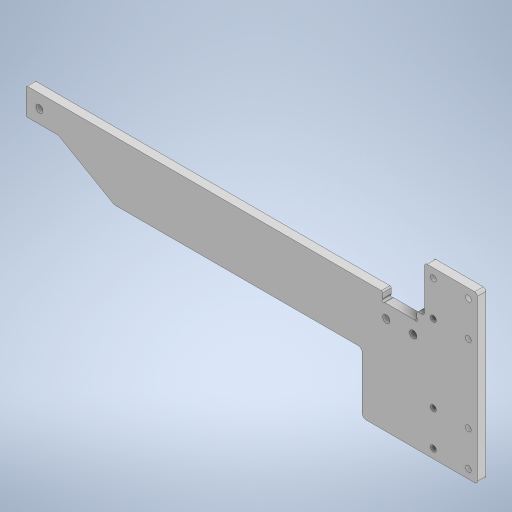
# Autodesk Inventor part: Z-Axis Bed Plates
Saved by Autodesk Inventor 2024 (Build 280153000, 153)
## iProperties
Created: 2024-08-02
Part Number: Z-Axis Bed Plates
Material: Generic
Document SubType Name: Modeling
Designer: Ishaan
Density: 1 g/cm^3
Appearance: Default
Author: Ishaan
Autodesk Inventor part; units mm, degrees
ref_plane "YZ Plane" through (0, 0, 0) normal (1, 0, 0) x (0, 1, 0)
ref_plane "XZ Plane" through (0, 0, 0) normal (0, 1, 0) x (-1, 0, 0)
sketch "Sketch1" plane through (0, 0, 0) normal (0, 0, 1) x (1, 0, 0)
  line L0 (19.7, -72.5) -> (-19.7, -72.5)
  line L1 (-19.7, -72.5) -> (-19.7, 72.5)
  line L2 (-19.7, 72.5) -> (19.7, 72.5)
  line L3 (19.7, 72.5) -> (19.7, -72.5)
  line L4 (19.7, -72.5) -> (-19.7, 72.5) construction
  line L5 (-19.7, -72.5) -> (19.7, 72.5) construction
  line L6 (19.7, 11.1) -> (-19.7, 11.1) construction
  line L7 (-19.7, 11.1) -> (-19.7, 72.5) construction
  line L8 (-19.7, 72.5) -> (19.7, 72.5) construction
  line L9 (19.7, 72.5) -> (19.7, 11.1) construction
  line L10 (19.7, 11.1) -> (-19.7, 72.5) construction
  line L11 (-19.7, 11.1) -> (19.7, 72.5) construction
  line L12 (19.7, -72.5) -> (-19.7, -72.5) construction
  line L13 (-19.7, -72.5) -> (-19.7, -11.1) construction
  line L14 (-19.7, -11.1) -> (19.7, -11.1) construction
  line L15 (19.7, -11.1) -> (19.7, -72.5) construction
  line L16 (19.7, -72.5) -> (-19.7, -11.1) construction
  line L17 (-19.7, -72.5) -> (19.7, -11.1) construction
  line L18 (19.7, 22.1) -> (-19.7, 22.1) construction
  line L19 (-19.7, 22.1) -> (-19.7, 61.5) construction
  line L20 (-19.7, 61.5) -> (19.7, 61.5)
  line L21 (19.7, 61.5) -> (19.7, 22.1) construction
  line L22 (19.7, 22.1) -> (-19.7, 61.5) construction
  line L23 (-19.7, 22.1) -> (19.7, 61.5) construction
  line L24 (19.7, -61.5) -> (-19.7, -61.5)
  line L25 (-19.7, -61.5) -> (-19.7, -22.1) construction
  line L26 (-19.7, -22.1) -> (19.7, -22.1) construction
  line L27 (19.7, -22.1) -> (19.7, -61.5) construction
  line L28 (19.7, -61.5) -> (-19.7, -22.1) construction
  line L29 (-19.7, -61.5) -> (19.7, -22.1) construction
  line L30 (13, 28.8) -> (-13, 28.8) construction
  line L31 (-13, 28.8) -> (-13, 54.8) construction
  line L32 (-13, 54.8) -> (13, 54.8) construction
  line L33 (13, 54.8) -> (13, 28.8) construction
  line L34 (13, 28.8) -> (-13, 54.8) construction
  line L35 (-13, 28.8) -> (13, 54.8) construction
  line L36 (13, -54.8) -> (-13, -54.8) construction
  line L37 (-13, -54.8) -> (-13, -28.8) construction
  line L38 (-13, -28.8) -> (13, -28.8) construction
  line L39 (13, -28.8) -> (13, -54.8) construction
  line L40 (13, -54.8) -> (-13, -28.8) construction
  line L41 (-13, -54.8) -> (13, -28.8) construction
  line L42 (-316, 27.5) -> (-19.7, 27.5)
  line L43 (-19.7, 27.5) -> (-19.7, 7.5)
  line L44 (-19.7, 7.5) -> (-316, 7.5)
  line L45 (-316, 7.5) -> (-316, 27.5)
  line L46 (19.7, -63.5) -> (19.7, -63.5)
  line L47 (19.772, 73.498) -> (19.772, 73.498)
  point P0 (0, 0)
  point P1 (0, 41.8)
  point P2 (0, -41.8)
  point P3 (-316, 17.5)
  point P4 (-291, 7.5)
  point P5 (17, 72.5)
  point P6 (17, -72.5)
  point P7 (-19.7, 27.5)
  point P8 (-19.7, 7.5)
  point P9 (-19.7, -61.5)
  point P10 (19.7, -61.5)
  dimension "d1" = 145
  dimension "d2" = 61.4
  dimension "d3" = 39.4
  dimension "d4" = 26
  dimension "d5" = 26
  dimension "d6" = 20
  dimension "d8" = 316
  dimension "d11" = 25
  dimension "d55" = 45
  dimension "d126" = 6.7
  dimension "d128" = 6.7
  constraints: 96 end point, 17 parallel, 15 midpoint, 9 collinear, 9 horizontal, 8 coincident, 8 perpendicular, 4 equal length, 2 point on line
  measures "d1" distance between parallel lines of L2 L0
  measures "d2" distance of L6.end L7.end
  measures "d3" distance of L18.end L19.end
  measures "d4" distance of L31.end L32.end
  measures "d5" distance of L30.end L31.end
  measures "d6" distance of L44.end L42.start
  measures "d8" distance from line of point (0, 41.8) L45
  measures "d11" distance from line of point (-291, 7.5) L45
  measures "d55" distance between parallel lines of L2 L42
  measures "d126" distance from line of L20 point (13, 54.8)
  measures "d128" distance between parallel lines of L21 L33
extrude "Extrusion1" add sketch "Sketch1" along normal blind 6.35 contours L24 L1 L20 L3 | L44 L45 L42 L1
sketch "Sketch2" plane through (0, 0, 6.35) normal (0, 0, 1) x (1, 0, 0)
  line L0 (19.7, -61.5) -> (19.7, 61.5) projected
  line L1 (-19.7, 61.5) -> (-19.7, 27.5) projected
  line L2 (-19.7, 27.5) -> (-316, 27.5) projected
  line L3 (-316, 27.5) -> (-316, 7.5) projected
  line L4 (-316, 7.5) -> (-19.7, 7.5) projected
  line L5 (-19.7, 7.5) -> (-19.7, -61.5) projected
  line L6 (19.7, -61.5) -> (-19.7, -61.5) construction
  line L7 (-19.7, -61.5) -> (19.7, -61.5) projected
  line L8 (19.7, 61.5) -> (-19.7, 61.5) projected
  line L9 (-19.7, -61.5) -> (-66, -61.5)
  line L10 (-66, -16.5) -> (-250.4308, -16.5)
  line L11 (-250.4308, -16.5) -> (-292, 7.5)
  line L12 (-66, -16.5) -> (-66, -61.5)
  point P0 (0, 0)
  point P1 (0, 41.8)
  point P2 (0, -41.8)
  point P3 (13, 28.8)
  point P4 (13, -28.8)
  dimension "d25" = 24
  dimension "d124" = 34
  dimension "d140" = 24
  dimension "d142" = 85.7
  dimension "d143" = 150
  constraints: 8 end point, 2 horizontal, 2 point on line, 1 collinear, 1 parallel
  measures "d25" distance from line of L11.end L3
  measures "d124" distance between parallel lines of L8 L2
  measures "d140" distance between parallel lines of L10 L4
  measures "d142" distance from line of L0 L9.end
  measures "d143" angle of L10 L11
extrude "Extrusion2" add sketch "Sketch2" against normal up to surface (6.35 mm away) contours L9 L12 L10 L11 L4 L5
hole "Hole1" at (-13, 54.8, 0) at (13, 54.8, 0) at (13, 28.8, 0) at (-13, 28.8, 0) at (-13, -28.8, 0) at (13, -28.8, 0) at (13, -54.8, 0) at (-13, -54.8, 0) direction (0, 0, 1) diameter 4.2 end through all
sketch "Z POSITIONING" plane through (0, 0, 6.35) normal (0, 0, 1) x (1, 0, 0)
  circle A0 centre (-13, -54.8) radius 2.1 projected
  circle A1 centre (13, -54.8) radius 2.1 projected
  circle A2 centre (13, -28.8) radius 2.1 projected
  circle A3 centre (-13, -28.8) radius 2.1 projected
  circle A4 centre (-13, 28.8) radius 2.1 projected
  circle A5 centre (13, 28.8) radius 2.1 projected
  circle A6 centre (13, 54.8) radius 2.1 projected
  circle A7 centre (-13, 54.8) radius 2.1 projected
  line L0 (-19.7, 27.5) -> (-316, 27.5) projected
  line L1 (-316, 27.5) -> (-316, 7.5) projected
  line L2 (-316, 7.5) -> (-292, 7.5) projected
  line L3 (-73.0306, 76.9979) -> (-73.0306, 70.6479)
  line L4 (-13, 54.8) -> (13, 54.8) construction
  line L5 (-51.9212, 35.5) -> (-16.9212, 35.5) construction
  line L6 (-16.9212, 35.5) -> (-16.9212, 27.5) construction
  line L7 (-16.9212, 27.5) -> (-51.9212, 27.5) construction
  line L8 (-51.9212, 27.5) -> (-51.9212, 35.5) construction
  line L9 (-51.9212, 69.65) -> (-6.1684, 69.65) construction
  line L10 (-125.0107, 76) -> (3.0638, 76) construction
  line L11 (3.0638, 76) -> (3.0638, 69.65) construction
  line L12 (3.0638, 69.65) -> (-125.0107, 69.65) construction
  line L13 (-125.0107, 69.65) -> (-125.0107, 76) construction
  line L14 (-120.28, 89) -> (-45.2895, 89) construction
  line L15 (-45.2895, 89) -> (-45.2895, 76) construction
  line L16 (-45.2895, 76) -> (-120.28, 76) construction
  line L17 (-120.28, 76) -> (-120.28, 89) construction
  line L18 (-46.2871, 30.7481) -> (-33.7765, 30.7481) construction
  line L19 (-33.7765, 30.7481) -> (-33.7765, 27.5) construction
  line L20 (-33.7765, 27.5) -> (-46.2871, 27.5) construction
  line L21 (-46.2871, 27.5) -> (-46.2871, 30.7481) construction
  line L22 (-83.6356, 76.3105) -> (-20.2105, 76.3105) construction
  line L23 (-20.2105, 76.3105) -> (-20.2105, 72.407) construction
  line L24 (-20.2105, 72.407) -> (-83.6356, 72.407) construction
  line L25 (-83.6356, 72.407) -> (-83.6356, 76.3105) construction
  line L26 (-72.5883, 73.6984) -> (-50.3384, 73.6984) construction
  line L27 (-50.3384, 73.6984) -> (-50.3384, 69.65) construction
  line L28 (-50.3384, 69.65) -> (-72.5883, 69.65) construction
  line L29 (-72.5883, 69.65) -> (-72.5883, 73.6984) construction
  line L30 (-111.3546, 80.0484) -> (-73.1953, 80.0484) construction
  line L31 (-73.1953, 80.0484) -> (-73.1953, 76) construction
  line L32 (-73.1953, 76) -> (-111.3546, 76) construction
  line L33 (-111.3546, 76) -> (-111.3546, 80.0484) construction
  line L34 (-122.3616, 95.35) -> (-60.8324, 95.35) construction
  line L35 (-60.8324, 95.35) -> (-60.8324, 89) construction
  line L36 (-60.8324, 89) -> (-122.3616, 89) construction
  line L37 (-122.3616, 89) -> (-122.3616, 95.35) construction
  line L38 (-97.4496, 108.35) -> (-64.4997, 108.35) construction
  line L39 (-64.4997, 108.35) -> (-64.4997, 95.35) construction
  line L40 (-64.4997, 95.35) -> (-97.4496, 95.35) construction
  line L41 (-97.4496, 95.35) -> (-97.4496, 108.35) construction
  line L42 (-105.6043, 93.0261) -> (-84.5103, 93.0261) construction
  line L43 (-84.5103, 93.0261) -> (-84.5103, 89) construction
  line L44 (-84.5103, 89) -> (-105.6043, 89) construction
  line L45 (-105.6043, 89) -> (-105.6043, 93.0261) construction
  line L46 (-109.4941, 99.3984) -> (-71.3471, 99.3984) construction
  line L47 (-71.3471, 99.3984) -> (-71.3471, 95.35) construction
  line L48 (-71.3471, 95.35) -> (-109.4941, 95.35) construction
  line L49 (-109.4941, 95.35) -> (-109.4941, 99.3984) construction
  line L50 (-134.6087, 111.525) -> (-34.6087, 111.525) construction
  line L51 (-34.6087, 111.525) -> (-34.6087, 108.35) construction
  line L52 (-34.6087, 108.35) -> (-134.6087, 108.35) construction
  line L53 (-134.6087, 108.35) -> (-134.6087, 111.525) construction
  line L54 (-97.1464, 115.5511) -> (-69.166, 115.5511) construction
  line L55 (-69.166, 115.5511) -> (-69.166, 111.525) construction
  line L56 (-69.166, 111.525) -> (-97.1464, 111.525) construction
  line L57 (-97.1464, 111.525) -> (-97.1464, 115.5511) construction
  line L58 (-143.7669, 61.65) -> (-108.5896, 61.65) construction
  line L59 (-148.1315, 61.65) -> (-115.878, 61.65) construction
  line L60 (-115.878, 61.65) -> (-115.878, 58.4884) construction
  line L61 (-115.878, 58.4884) -> (-148.1315, 58.4884) construction
  line L62 (-148.1315, 58.4884) -> (-148.1315, 61.65) construction
  line L63 (-66, -61.5) -> (19.7, -61.5) projected
  line L64 (-19.7, 61.5) -> (-19.7, 27.5) projected
  line L65 (19.7, -61.5) -> (19.7, 61.5) projected
  line L66 (19.7, 61.5) -> (-19.7, 61.5) projected
  line L67 (-292, 7.5) -> (-250.4308, -16.5) projected
  line L68 (-250.4308, -16.5) -> (-66, -16.5) projected
  line L69 (-66, -16.5) -> (-66, -61.5) projected
  point P0 (0, 0)
  point P1 (0, 54.8)
  dimension "d39" = 6.35
  dimension "d42" = 35
  dimension "d43" = 8
  dimension "d44" = 34.15
  dimension "d45" = 6.35
  dimension "d46" = 13
  dimension "d48" = 6.35
  dimension "d49" = 13
  dimension "d50" = 100
  dimension "d51" = 3.175
  dimension "d52" = 46.7
  dimension "d53" = 34.15
  constraints: 56 end point, 13 collinear, 12 parallel, 9 horizontal, 6 perpendicular, 1 midpoint, 16 other
  measures "d39" distance of L3.start L3.end
  measures "d42" distance of L6.end L7.end
  measures "d43" distance of L5.end L6.end
  measures "d44" distance between parallel lines of L5 L9
  measures "d45" distance of L10.end L11.end
  measures "d46" distance of L14.end L15.end
  measures "d48" distance of L34.end L35.end
  measures "d49" distance of L38.end L39.end
  measures "d50" distance of L51.end L52.end
  measures "d51" distance of L50.end L51.end
  measures "d52" distance between parallel lines of L52 L58
  measures "d53" distance between parallel lines of L0 L58
ref_plane "PRINTBED PLANE" through (-316, 61.65, 6.35) normal (0, 1, 0) x (1, 0, 0)
sketch "Y POSITIONING" plane through (0, 0, 6.35) normal (0, 0, 1) x (1, 0, 0)
  line L0 (-315, 61.65) -> (-29, 61.65) construction
  line L1 (-306, 61.65) -> (-306, 54.4706) construction
  line L2 (-38, 61.65) -> (-38, 46.65) construction
  line L3 (-316, 27.5) -> (-316, 7.5) projected
  line L4 (-32, 27.5) -> (-44, 27.5) construction
  line L5 (-44, 27.5) -> (-44, 61.65) construction
  line L6 (-44, 61.65) -> (-32, 61.65) construction
  line L7 (-32, 61.65) -> (-32, 27.5) construction
  line L8 (-32, 27.5) -> (-44, 61.65) construction
  line L9 (-44, 27.5) -> (-32, 61.65) construction
  line L10 (-19.7, 27.5) -> (-316, 27.5) projected
  circle A0 centre (-13, -54.8) radius 2.1 projected
  circle A1 centre (13, -54.8) radius 2.1 projected
  circle A2 centre (13, -28.8) radius 2.1 projected
  circle A3 centre (-13, -28.8) radius 2.1 projected
  circle A4 centre (-13, 28.8) radius 2.1 projected
  circle A5 centre (13, 28.8) radius 2.1 projected
  circle A6 centre (13, 54.8) radius 2.1 projected
  circle A7 centre (-13, 54.8) radius 2.1 projected
  line L11 (-19.7, 27.5) -> (-316, 27.5) projected
  line L12 (-316, 27.5) -> (-316, 7.5) projected
  line L13 (-316, 7.5) -> (-292, 7.5) projected
  line L14 (-13, 54.8) -> (13, 28.8) construction
  line L15 (-383.14, 61.65) -> (86.84, 61.65) construction
  line L16 (-53, 27.5) -> (-23, 27.5) construction
  line L17 (-23, 27.5) -> (-23, 35.5) construction
  line L18 (-23, 35.5) -> (-53, 35.5) construction
  line L19 (-53, 35.5) -> (-53, 27.5) construction
  line L20 (-53, 27.5) -> (-23, 35.5) construction
  line L21 (-23, 27.5) -> (-53, 35.5) construction
  line L22 (-66, -61.5) -> (19.7, -61.5) projected
  line L23 (-58, 21.15) -> (-18, 21.15) construction
  line L24 (-18, 21.15) -> (-18, 1.15) construction
  line L25 (-18, 1.15) -> (-58, 1.15) construction
  line L26 (-58, 1.15) -> (-58, 21.15) construction
  line L27 (-48, 11.15) -> (-28, 11.15) construction
  line L28 (-19.7, 61.5) -> (-19.7, 27.5) projected
  line L29 (19.7, -61.5) -> (19.7, 61.5) projected
  line L30 (19.7, 61.5) -> (-19.7, 61.5) projected
  line L31 (-292, 7.5) -> (-250.4308, -16.5) projected
  line L32 (-250.4308, -16.5) -> (-66, -16.5) projected
  line L33 (-66, -16.5) -> (-66, -61.5) projected
  point P0 (0, 0)
  point P1 (-38, 44.575)
  point P2 (-32, 47.5)
  point P3 (0, 41.8)
  point P4 (-38, 31.5)
  point P5 (-38, 27.5)
  point P6 (-38, 21.15)
  point P7 (-38, 11.15)
  point P8 (-18, 11.15)
  dimension "d58" = 286
  dimension "d60" = 9
  dimension "d61" = 10
  dimension "d62" = 12
  dimension "d63" = 38
  dimension "d64" = 9
  dimension "d65" = 30
  dimension "d66" = 8
  dimension "d67" = 15
  dimension "d68" = 19.15
  dimension "d83" = 40
  dimension "d84" = 20
  dimension "d85" = 6.35
  dimension "d90" = 20
  constraints: 42 end point, 10 midpoint, 6 horizontal, 6 parallel, 4 point on line, 3 perpendicular, 2 coincident, 2 collinear, 2 vertical, 1 vertical alignment, 1 other
  measures "d58" distance of L0.start L0.end
  measures "d60" distance from line of L0.end L2
  measures "d61" distance between parallel lines of L1 L3
  measures "d62" distance between parallel lines of L7 L5
  measures "d63" horizontal distance of point (-38, 44.575) point (0, 41.8)
  measures "d64" distance from line of L1 L0.start
  measures "d65" distance of L17.end L18.end
  measures "d66" distance of L16.end L17.end
  measures "d67" distance from line of L2.end L15
  measures "d83" distance of L24.end L25.end
  measures "d84" distance of L23.end L24.end
  measures "d90" distance of L27.start L27.end
sketch "Sketch5" plane through (0, 0, 6.35) normal (0, 0, 1) x (1, 0, 0)
  line L0 (-296, 7.5) -> (-316, 7.5) construction
  line L1 (-316, 7.5) -> (-316, 27.5) construction
  line L2 (-316, 27.5) -> (-296, 27.5) construction
  line L3 (-296, 27.5) -> (-296, 7.5) construction
  line L4 (-296, 7.5) -> (-316, 27.5) construction
  line L5 (-316, 7.5) -> (-296, 27.5) construction
  point P0 (0, 0)
  point P1 (-306, 17.5)
  point P2 (-306, 17.5)
  constraints: 12 end point, 3 coincident, 2 midpoint, 2 parallel, 2 perpendicular, 1 horizontal
hole "Hole2" at (-306, 17.5, 6.35) direction (0, 0, -1) diameter 5.2 end through all
sketch "Sketch6" plane through (0, 0, 6.35) normal (0, 0, 1) x (1, 0, 0)
  line L0 (-50.75, 27.5) -> (-25.25, 27.5)
  line L1 (-25.25, 27.5) -> (-25.25, 21.15)
  line L2 (-25.25, 21.15) -> (-50.75, 21.15)
  line L3 (-50.75, 21.15) -> (-50.75, 27.5)
  line L4 (-38, 61.65) -> (-38, 46.65) construction
  line L5 (-19.7, 27.5) -> (-316, 27.5) projected
  line L6 (-58, 21.15) -> (-18, 21.15) construction
  circle A0 centre (-50.25, 21.65) radius 0.875
  circle A1 centre (-25.75, 21.65) radius 0.875
  point P0 (0, 0)
  point P1 (-38, 27.5)
  point P2 (-32, 47.5)
  point P3 (-26.4681, 21.15)
  point P4 (-25.25, 22.3681)
  point P5 (-50.75, 22.3681)
  point P6 (-49.5319, 21.15)
  dimension "d79" = 25.5
  dimension "d86" = 1.75
  dimension "d87" = 0.5
  dimension "d88" = 0.5
  dimension "d89" = 0.5
  constraints: 8 end point, 2 centre point, 2 horizontal, 2 parallel, 1 collinear, 1 equal radius, 1 horizontal alignment, 1 midpoint, 1 perpendicular, 1 point on line, 1 other
  measures "d79" distance of L1.end L2.end
  measures "d86" diameter of A0
  measures "d87" distance from line of L2 A0.centre
  measures "d88" distance from line of A0.centre L3
  measures "d89" distance from line of L1 A1.centre
extrude "Extrusion3" cut sketch "Sketch6" against normal through all
hole "Hole3" at (-48, 11.15, 6.35) at (-28, 11.15, 6.35) direction (0, 0, -1) diameter 5.3 end through all
sketch "Sketch9" plane through (0, 0, 6.35) normal (0, 0, 1) x (1, 0, 0)
  circle A0 centre (-28, 11.15) radius 2.65 projected
  circle A1 centre (-48, 11.15) radius 2.65 projected
  line L0 (-50.75, 22.3681) -> (-50.75, 27.5) projected
  line L1 (-50.75, 27.5) -> (-316, 27.5) projected
  line L2 (-316, 27.5) -> (-316, 7.5) projected
  line L3 (-316, 7.5) -> (-292, 7.5) projected
  line L4 (-66, -61.5) -> (19.7, -61.5) projected
  line L5 (-25.25, 27.5) -> (-25.25, 22.3681) projected
  arc A2 (-26.4681, 21.15) -> (-25.25, 22.3681) centre (-25.75, 21.65) ccw projected
  line L6 (-26.4681, 21.15) -> (-49.5319, 21.15) projected
  arc A3 (-50.75, 22.3681) -> (-49.5319, 21.15) centre (-50.25, 21.65) ccw projected
  circle A4 centre (-306, 17.5) radius 2.6 projected
  circle A5 centre (-13, -54.8) radius 2.1 projected
  circle A6 centre (13, -54.8) radius 2.1 projected
  circle A7 centre (13, -28.8) radius 2.1 projected
  circle A8 centre (-13, -28.8) radius 2.1 projected
  circle A9 centre (-13, 28.8) radius 2.1 projected
  circle A10 centre (13, 28.8) radius 2.1 projected
  circle A11 centre (13, 54.8) radius 2.1 projected
  circle A12 centre (-13, 54.8) radius 2.1 projected
  line L7 (-19.7, 61.5) -> (-19.7, 27.5) projected
  line L8 (19.7, -61.5) -> (19.7, 61.5) projected
  line L9 (19.7, 61.5) -> (-19.7, 61.5) projected
  line L10 (-19.7, 27.5) -> (-25.25, 27.5) projected
  line L11 (-292, 7.5) -> (-250.4308, -16.5) projected
  line L12 (-250.4308, -16.5) -> (-66, -16.5) projected
  line L13 (-66, -16.5) -> (-66, -61.5) projected
  point P0 (0, 0)
fillet "Fillet3" radius 1 8 edges at (-316, 27.5, 3.175) (-316, 7.5, 3.175) (-50.75, 27.5, 3.175) (-50.75, 22.3681, 3.175) (-49.5319, 21.15, 3.175) (-26.4681, 21.15, 3.175) (-25.25, 22.3681, 3.175) (-25.25, 27.5, 3.175)
fillet "Fillet4" radius 3 4 edges at (-66, -61.5, 3.175) (-250.4308, -16.5, 3.175) (-66, -16.5, 3.175) (-292, 7.5, 3.175)
fillet "Fillet5" radius 2 4 edges at (-19.7, 27.5, 3.175) (-19.7, 61.5, 3.175) (19.7, 61.5, 3.175) (19.7, -61.5, 3.175)
sketch "Sketch10" plane through (0, 0, 6.35) normal (0, 0, 1) x (1, 0, 0)
  line L0 (-163.15, 17.9395) -> (-148.15, 26.5998)
  line L1 (-148.15, 26.5998) -> (-133.15, 17.9395)
  line L2 (-133.15, 17.9395) -> (-133.15, 0.619)
  line L3 (-133.15, 0.619) -> (-148.15, -8.0412)
  line L4 (-148.15, -8.0412) -> (-163.15, 0.619)
  line L5 (-163.15, 0.619) -> (-163.15, 17.9395)
  arc A0 (17.7, -59) -> (19.7, -57) centre (17.7, -57) ccw projected
  line L6 (19.7, -57) -> (19.7, 57) projected
  arc A1 (19.7, 57) -> (17.7, 59) centre (17.7, 57) ccw projected
  line L7 (17.7, 59) -> (-17.7, 59) projected
  arc A2 (-17.7, 59) -> (-19.7, 57) centre (-17.7, 57) ccw projected
  line L8 (-19.7, 57) -> (-19.7, 42) projected
  arc A3 (-21.7, 40) -> (-19.7, 42) centre (-21.7, 42) ccw projected
  line L9 (-21.7, 40) -> (-24.25, 40) projected
  arc A4 (-24.25, 40) -> (-25.25, 39) centre (-24.25, 39) ccw projected
  line L10 (-25.25, 39) -> (-25.25, 35.275) projected
  arc A5 (-25.25, 35.275) -> (-25.05, 34.675) centre (-24.25, 35.275) ccw projected
  arc A6 (-26.275, 33.45) -> (-25.05, 34.675) centre (-25.75, 34.15) ccw projected
  arc A7 (-26.275, 33.45) -> (-26.875, 33.65) centre (-26.875, 32.65) ccw projected
  line L11 (-26.875, 33.65) -> (-49.125, 33.65) projected
  arc A8 (-49.125, 33.65) -> (-49.725, 33.45) centre (-49.125, 32.65) ccw projected
  arc A9 (-50.95, 34.675) -> (-49.725, 33.45) centre (-50.25, 34.15) ccw projected
  arc A10 (-50.95, 34.675) -> (-50.75, 35.275) centre (-51.75, 35.275) ccw projected
  line L12 (-50.75, 35.275) -> (-50.75, 39) projected
  arc A11 (-50.75, 39) -> (-51.75, 27.5) centre (-51.75, 39) ccw projected
  line L13 (-51.75, 40) -> (-315, 40) projected
  arc A12 (-315, 27.5) -> (-316, 39) centre (-315, 39) ccw projected
  line L14 (-316, 39) -> (-316, 21) projected
  arc A13 (-316, 21) -> (-315, 20) centre (-315, 21) ccw projected
  line L15 (-315, 20) -> (-301.6658, 20) projected
  arc A14 (-300.3574, 19.8258) -> (-301.6658, 20) centre (-301.6658, 15) ccw projected
  line L16 (-300.3574, 19.8258) -> (-80.3426, -39.8258) projected
  arc A15 (-80.3426, -39.8258) -> (-79.0342, -40) centre (-79.0342, -35) ccw projected
  line L17 (-79.0342, -40) -> (-21.7, -40) projected
  arc A16 (-19.7, -42) -> (-21.7, -40) centre (-21.7, -42) ccw projected
  line L18 (-19.7, -42) -> (-19.7, -57) projected
  arc A17 (-19.7, -57) -> (-17.7, -59) centre (-17.7, -57) ccw projected
  line L19 (-17.7, -59) -> (17.7, -59) projected
  circle A18 centre (-28, 23.65) radius 2.65 projected
  circle A19 centre (-48, 23.65) radius 2.65 projected
  circle A20 centre (-306, 30) radius 2.6 projected
  circle A21 centre (-13, -52.3) radius 2.1 projected
  circle A22 centre (13, -52.3) radius 2.1 projected
  circle A23 centre (13, -26.3) radius 2.1 projected
  circle A24 centre (-13, -26.3) radius 2.1 projected
  circle A25 centre (-13, 26.3) radius 2.1 projected
  circle A26 centre (13, 26.3) radius 2.1 projected
  circle A27 centre (13, 52.3) radius 2.1 projected
  circle A28 centre (-13, 52.3) radius 2.1 projected
  line L20 (-163.15, 17.9395) -> (-148.15, 9.2793)
  line L21 (-148.15, 9.2793) -> (-133.15, 17.9395)
  line L22 (-148.15, 9.2793) -> (-148.15, -8.0412) construction
  line L23 (-148.15, 0.619) -> (-163.15, 9.2793)
  line L24 (-148.15, 0.619) -> (-133.15, 9.2793)
  line L25 (-133.15, 15.0528) -> (-148.15, 6.3925)
  line L26 (-148.15, 6.3925) -> (-163.15, 15.0528)
  line L27 (-163.15, 6.3925) -> (-148.15, -2.2677)
  line L28 (-148.15, -2.2677) -> (-133.15, 6.3925)
  line L29 (-51.75, 27.5) -> (-315, 27.5) construction
  line L30 (-148.15, 40) -> (-148.15, -21.4415) construction
  line L31 (-316, 30) -> (19.7, 30) construction
  point P0 (0, 0)
  point P1 (-148.15, 30)
  dimension "d132" = 30
  dimension "d133" = 5
  dimension "d134" = 2.5
  dimension "d135" = 5
  constraints: 34 end point, 8 point on line, 6 midpoint, 4 parallel, 3 vertical, 1 coincident, 1 collinear, 1 perpendicular, 1 vertical alignment, 17 other
  measures "d132" distance between parallel lines of L2 L5
  measures "d133" distance between parallel lines of L3 L28
  measures "d134" distance between parallel lines of L28 L24
  measures "d135" distance between parallel lines of L24 L25
equation "\"d54\" = d53"
body "Solid1"
